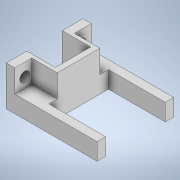
# Autodesk Inventor part: Bracket motoren
Saved by Autodesk Inventor 2022 (Build 260153000, 153)
## iProperties
Created: 2022-10-14
Part Number: Bracket motoren
Material: Generic
Document SubType Name: Modeling
Designer: Kilian De Ruyck
Density: 1 g/cm^3
Appearance: Default
Author: Kilian De Ruyck
Autodesk Inventor part; units mm, degrees
ref_plane "YZ Plane" through (0, 0, 0) normal (1, 0, 0) x (0, 1, 0)
ref_plane "XZ Plane" through (0, 0, 0) normal (0, 1, 0) x (-1, 0, 0)
sketch "Sketch2" plane through (0, 0, 0) normal (0, 1, 0) x (-1, 0, 0)
  line L0 (0, 0) -> (-10.5, 0)
  line L1 (-10.5, 0) -> (-10.5, -12.5)
  line L2 (-10.5, -12.5) -> (0, -12.5)
  line L3 (0, -12.5) -> (0, 0)
  line L4 (0, 0) -> (0, 1.25)
  line L5 (0, 1.25) -> (-12, 1.25)
  line L6 (-12, 1.25) -> (-12, -13.75)
  line L7 (-12, -13.75) -> (0, -13.75)
  line L8 (0, -13.75) -> (0, -12.5)
  dimension "d8" = 10.5
  dimension "d9" = 12.5
  dimension "d10" = 1.25
  dimension "d11" = 12
  dimension "d12" = 15
  constraints: 18 end point, 4 perpendicular, 2 parallel, 1 collinear, 1 horizontal, 1 point on line, 1 vertical
  measures "d8" distance of L2.end L1.end
  measures "d9" distance of L1.end L0.end
  measures "d10" distance of L0.start L4.end
  measures "d11" distance of L4.end L5.end
  measures "d12" distance of L5.end L6.end
extrude "Extrusion2" add sketch "Sketch2" along normal blind 9 contours L0 L1 L2 L8 L7 L6 L5 L4
ref_plane "Work Plane1" through (2, 0, 0) normal (-1, 0, 0) x (0, 0, 1)
sketch "Sketch9" plane through (0, 9, 0) normal (-1, 0, 0) x (0, 0, 1)
  line L0 (1.25, -9) -> (1.25, 0) projected
  line L1 (1.25, -9) -> (7.25, -9)
  line L2 (7.25, -9) -> (7.25, 0)
  line L3 (7.25, 0) -> (1.25, 0)
  line L4 (1.25, 0) -> (1.25, -9)
  line L5 (-13.75, -9) -> (-13.75, 0) projected
  line L6 (-13.75, 0) -> (-19.75, 0)
  line L7 (-19.75, 0) -> (-19.75, -9)
  line L8 (-19.75, -9) -> (-13.75, -9)
  line L9 (-13.75, -9) -> (-13.75, 0)
  point P0 (0, -9)
  dimension "d67" = 6
  dimension "d68" = 6
  dimension "d69" = 9
  constraints: 16 end point, 4 parallel, 2 horizontal, 2 perpendicular
  measures "d67" distance of L3.end L2.end
  measures "d68" distance of L8.end L7.end
  measures "d69" distance of L7.end L6.end
extrude "Extrusion6" add sketch "Sketch9" against normal blind 3
sketch "Sketch11" plane through (3, 9, 0) normal (1, 0, 0) x (0, 0, -1)
  line L0 (-1.25, 0) -> (-7.25, 0) projected
  line L1 (-7.25, 0) -> (-7.25, -9) projected
  line L2 (19.75, -9) -> (19.75, 0) projected
  line L3 (19.75, 0) -> (13.75, 0) projected
  point P0 (0, -9)
  point P1 (-3.75, -4.5)
  point P2 (16.25, -4.5)
  dimension "d83" = 4.5
  dimension "d84" = 3.5
  dimension "d85" = 3.5
  dimension "d86" = 4.5
  measures "d83" distance from line of L0 point (-3.75, -4.5)
  measures "d84" distance from line of L1 point (-3.75, -4.5)
  measures "d85" distance from line of L2 point (16.25, -4.5)
  measures "d86" distance from line of L3 point (16.25, -4.5)
hole "Hole4" at (3, 4.5, 3.75) at (3, 4.5, -16.25) direction (-1, 0, 0) diameter 3.5 depth 3
sketch "Sketch12" plane through (10.5, 0, -12.5) normal (-1, 0, 0) x (0, 0, 1)
  line L0 (12.5, 0) -> (12.5, 9) projected
  line L1 (0, 0) -> (0, 9) projected
  line L2 (12.5, 9) -> (0, 9)
  line L3 (0, 9) -> (0, 0)
  line L4 (0, 0) -> (12.5, 0)
  line L5 (12.5, 0) -> (12.5, 9)
  line L6 (0, 9) -> (12.5, 9) projected
  dimension "d94" = 9
  dimension "d95" = 0
  constraints: 8 end point, 2 parallel, 2 point on line, 1 horizontal, 1 perpendicular
  measures "d94" distance of L3.end L2.end
  measures "d95" distance between parallel lines of L6 L2
extrude "Extrusion7" add sketch "Sketch12" along normal blind 0.5
sketch "Sketch13" plane through (0, 0, 0) normal (0, -1, 0) x (1, 0, 0)
  line L0 (0, 0) -> (0, 7.25) projected
  line L1 (0, 7.25) -> (3, 7.25)
  line L2 (3, 7.25) -> (3, 0)
  line L3 (3, 0) -> (0, 0)
  line L4 (0, 0) -> (0, 7.25)
  line L5 (3, 1.25) -> (12, 1.25) projected
  line L6 (3, 0) -> (12, 0)
  line L7 (12, 0) -> (12, 1.25)
  line L8 (12, 1.25) -> (3, 1.25)
  line L9 (3, 1.25) -> (3, 0)
  line L10 (12, 1.25) -> (12, -13.75) projected
  line L11 (10, 0) -> (0, 0) projected
  line L12 (12, -13.75) -> (10, -13.75)
  line L13 (10, -13.75) -> (10, 0)
  line L14 (10, 0) -> (12, 0)
  line L15 (12, 0) -> (12, -13.75)
  line L16 (3, -19.75) -> (3, -13.75) projected
  line L17 (0, -12.5) -> (10, -12.5) projected
  line L18 (3, -19.75) -> (0, -19.75)
  line L19 (0, -19.75) -> (0, -12.5)
  line L20 (0, -12.5) -> (3, -12.5)
  line L21 (3, -12.5) -> (3, -19.75)
  line L22 (3, -13.75) -> (10, -13.75)
  line L23 (10, -13.75) -> (10, -12.5)
  line L24 (10, -12.5) -> (3, -12.5)
  line L25 (3, -12.5) -> (3, -13.75)
  line L26 (3, 7.25) -> (3, 1.25) projected
  point P0 (3, 1.25)
  dimension "d100" = 0
  constraints: 40 end point, 10 parallel, 5 horizontal, 5 perpendicular, 2 point on line
  measures "d100" distance between parallel lines of L26 L2
extrude "Extrusion8" add sketch "Sketch13" along normal blind 5
sketch "Sketch14" plane through (12, 9, 1.25) normal (1, 0, 0) x (0, 0, -1)
  line L0 (0, 0) -> (0, -14) projected
  line L1 (0, -14) -> (-6, -14)
  line L2 (-6, -14) -> (-6, -8)
  line L3 (-6, -8) -> (0, -8)
  line L4 (0, -8) -> (0, -14)
  line L5 (15, -14) -> (15, 0) projected
  line L6 (15, -14) -> (21, -14)
  line L7 (21, -14) -> (21, -8)
  line L8 (21, -8) -> (15, -8)
  line L9 (15, -8) -> (15, -14)
  point P0 (1.25, -9)
  dimension "d101" = 6
  dimension "d102" = 6
  dimension "d103" = 6
  dimension "d104" = 6
  constraints: 16 end point, 4 parallel, 2 horizontal, 2 perpendicular
  measures "d101" distance of L2.end L3.end
  measures "d102" distance of L1.end L2.end
  measures "d103" distance of L8.end L7.end
  measures "d104" distance of L7.end L6.end
extrude "Extrusion9" add sketch "Sketch14" against normal blind 10
sketch "Sketch18" plane through (12, 9, 1.25) normal (1, 0, 0) x (0, 0, -1)
  line L0 (-6, -14) -> (1.25, -14) projected
  line L1 (-6, -14) -> (-3, -14)
  line L2 (-3, -14) -> (-3, -8)
  line L3 (-3, -8) -> (-6, -8)
  line L4 (-6, -8) -> (-6, -14)
  line L5 (21, -14) -> (21, -8) projected
  line L6 (21, -14) -> (18, -14)
  line L7 (18, -14) -> (18, -8)
  line L8 (18, -8) -> (21, -8)
  line L9 (21, -8) -> (21, -14)
  point P0 (1.25, -9)
  dimension "d119" = 3
  dimension "d120" = 6
  dimension "d121" = 3
  dimension "d122" = 6
  constraints: 16 end point, 4 parallel, 2 horizontal, 2 perpendicular
  measures "d119" distance of L3.end L2.end
  measures "d120" distance of L2.end L1.end
  measures "d121" distance of L7.end L8.end
  measures "d122" distance of L6.end L7.end
extrude "Extrusion12" add sketch "Sketch18" along normal blind 20
equation "\"d85\" = d84"
body "Solid2"
